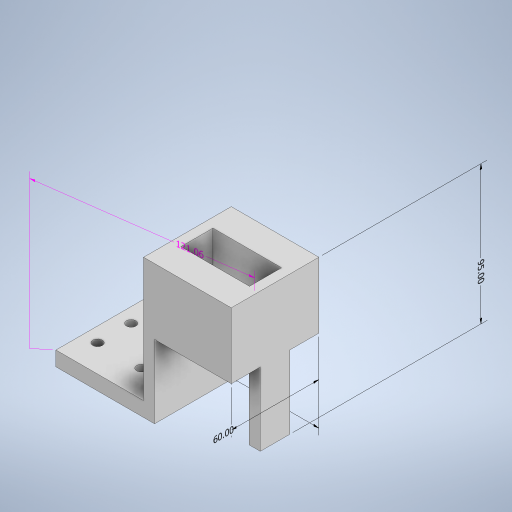
# Autodesk Inventor part: depth_camera_support_v2
Saved by Autodesk Inventor 2023 (Build 270158000, 158)
## iProperties
Created: 2023-05-27
Part Number: depth_camera_support_v2
Material: Genérico
Document SubType Name: Modeling
Designer: inigo
Density: 1 g/cm^3
Appearance: Valor por defecto
Author: inigo
Autodesk Inventor part; units mm, degrees
ref_plane "YZ Plane" through (0, 0, 0) normal (1, 0, 0) x (0, 1, 0)
ref_plane "XZ Plane" through (0, 0, 0) normal (0, 1, 0) x (-1, 0, 0)
ref_plane "XY Plane" through (0, 0, 0) normal (0, 0, 1) x (1, 0, 0)
sketch "Boceto2" plane through (0, 0, 0) normal (0, 1, 0) x (-1, 0, 0)
  line L0 (-30, 30) -> (30, 30)
  line L1 (30, 30) -> (30, -30)
  line L2 (30, -30) -> (-30, -30)
  line L3 (-30, -30) -> (-30, 30)
  line L4 (-30, 30) -> (30, -30) construction
  line L5 (30, 30) -> (-30, -30) construction
  point P0 (0, 0)
  dimension "d0" = 60
  dimension "d1" = 60
  constraints: 12 end point, 2 midpoint, 2 parallel, 1 horizontal, 1 perpendicular
  measures "d0" distance of L1.end L2.end
  measures "d1" distance of L0.end L1.end
extrude "Extrusión1" add sketch "Boceto2" along normal blind 55
sketch "Boceto3" plane through (30, 0, -30) normal (0, 0, -1) x (-1, 0, 0)
  line L0 (7.5, 50) -> (52.5, 50)
  line L1 (52.5, 50) -> (52.5, 0)
  line L2 (52.5, 0) -> (7.5, 0)
  line L3 (7.5, 0) -> (7.5, 50)
  line L4 (0, 0) -> (60, 0) projected
  point P0 (30, 0)
  dimension "d4" = 45
  dimension "d5" = 50
  dimension "d6" = 0
  constraints: 8 end point, 2 parallel, 1 horizontal, 1 perpendicular
  measures "d4" distance of L1.end L2.end
  measures "d5" distance of L0.end L1.end
  measures "d6" distance between parallel lines of L4 L2
extrude "Extrusión2" cut sketch "Boceto3" against normal blind 190
sketch "Boceto5" plane through (0, 0, 0) normal (0, 1, 0) x (-1, 0, 0)
  line L0 (30, -30) -> (30, 30) projected
  line L1 (30, 0) -> (60, 0)
  line L2 (90, 30) -> (30, 30)
  line L3 (30, 30) -> (30, -30)
  line L4 (30, -30) -> (90, -30)
  line L5 (90, -30) -> (90, 30)
  line L6 (90, 30) -> (30, -30) construction
  line L7 (30, 30) -> (90, -30) construction
  circle A0 centre (50, 11.5) radius 3.25
  circle A1 centre (50, -11.5) radius 3.25
  circle A2 centre (80, 11.5) radius 3.25
  circle A3 centre (80, -11.5) radius 3.25
  point P0 (0, 0)
  dimension "d16" = 30
  dimension "d17" = 60
  dimension "d18" = 60
  dimension "d19" = 6.5
  dimension "d20" = 20
  dimension "d21" = 18.5
  dimension "d22" = 23
  dimension "d23" = 6.5
  dimension "d24" = 30
  dimension "d25" = 18.5
  constraints: 14 end point, 4 centre point, 3 midpoint, 2 horizontal, 2 parallel, 2 symmetric about line, 1 perpendicular, 2 other
  measures "d16" distance of L1.start L1.end
  measures "d17" distance of L4.end L3.end
  measures "d18" distance of L3.end L2.end
  measures "d19" diameter of A0
  measures "d20" distance from line of L0 A0.centre
  measures "d21" distance from line of L2 A0.centre
  measures "d22" distance of A1.centre A0.centre
  measures "d23" diameter of A2
  measures "d24" distance of A0.centre A2.centre
  measures "d25" distance from line of L2 A2.centre
extrude "Extrusión4" add sketch "Boceto5" along normal blind 10
sketch "Boceto6" plane through (0, 55, 0) normal (0, 1, 0) x (1, 0, 0)
  line L0 (-30, 30) -> (-30, -30) projected
  line L1 (30, -30) -> (-30, -30)
  line L2 (-30, -30) -> (-30, 30)
  line L3 (-30, 30) -> (30, 30)
  line L4 (30, 30) -> (30, -30)
  line L5 (30, -30) -> (-30, 30) construction
  line L6 (-30, -30) -> (30, 30) construction
  point P0 (0, 0)
  dimension "d28" = 60
  constraints: 12 end point, 2 midpoint, 2 parallel, 1 horizontal, 1 perpendicular, 1 point on line
  measures "d28" distance of L1.end L2.end
extrude "Extrusión5" add sketch "Boceto6" along normal blind 40
sketch "Boceto7" plane through (0, 95, 0) normal (0, 1, 0) x (1, 0, 0)
  line L0 (-23.5, 11) -> (23.5, 11)
  line L1 (23.5, 11) -> (23.5, -11)
  line L2 (23.5, -11) -> (-23.5, -11)
  line L3 (-23.5, -11) -> (-23.5, 11)
  line L4 (-23.5, 11) -> (23.5, -11) construction
  line L5 (23.5, 11) -> (-23.5, -11) construction
  point P0 (0, 0)
  dimension "d31" = 47
  dimension "d32" = 22
  constraints: 12 end point, 2 midpoint, 2 parallel, 1 horizontal, 1 perpendicular
  measures "d31" distance of L1.end L2.end
  measures "d32" distance of L0.end L1.end
extrude "Extrusión6" cut sketch "Boceto7" against normal blind 43
sketch "Boceto8" plane through (-30, 0, 30) normal (-1, 0, 0) x (0, 0, 1)
  line L0 (-60, 55) -> (-44, 55) projected
  line L1 (0, 55) -> (-16, 55) projected
  line L2 (-44, 55) -> (-16, 55)
  line L3 (-41, 65) -> (-19, 65)
  line L4 (-19, 65) -> (-19, 55)
  line L5 (-19, 55) -> (-41, 55)
  line L6 (-41, 55) -> (-41, 65)
  line L7 (-41, 65) -> (-19, 55) construction
  line L8 (-19, 65) -> (-41, 55) construction
  line L9 (-16, 55) -> (-16, 95) projected
  line L10 (-44, 55) -> (-44, 95) projected
  point P0 (-30, 0)
  point P1 (-30, 60)
  point P2 (-41, 55)
  point P3 (-19, 55)
  point P4 (0, 95)
  point P5 (-60, 95)
  point P6 (-41, 60)
  dimension "d35" = 22
  dimension "d36" = 10
  dimension "d37" = 0
  dimension "d53" = 3
  dimension "d54" = 3
  constraints: 14 end point, 3 midpoint, 2 parallel, 1 collinear, 1 horizontal, 1 perpendicular
  measures "d35" distance of L4.end L5.end
  measures "d36" distance of L3.end L4.end
  measures "d37" distance between parallel lines of L5 L2
  measures "d53" distance between parallel lines of L9 L4
  measures "d54" distance from line of L10 point (-41, 60)
extrude "Extrusión7" cut sketch "Boceto8" against normal blind 10
ref_plane "Plano de trabajo1" through (30, 55, 0) normal (0, 0, -1) x (-1, 0, 0)
sketch "Boceto10" plane through (30, 55, 0) normal (0, 0, -1) x (-1, 0, 0)
  line L0 (60.12, -45) -> (60.12, 17.4198)
  line L1 (60.12, -45) -> (60.12, 13.5667)
  line L2 (60.12, -45) -> (137.1989, -45)
  line L3 (60.12, -19.9519) -> (80.5233, -61.6073)
  line L4 (120, -45) -> (60, -45) projected
  point P0 (30, -55)
  point P1 (72.3889, -45)
  dimension "d41" = 0
  constraints: 8 end point, 2 point on line
  measures "d41" distance between parallel lines of L4 L2
extrude "Extrusión8" add sketch "Boceto10" along normal mid plane 15
sketch "Boceto11" plane through (30, 0, 30) normal (1, 0, 0) x (0, 0, -1)
  line L0 (30, 0) -> (30, 50)
  line L1 (60, 50) -> (0, 50) projected
  line L2 (0, 0) -> (60, 0) projected
  line L3 (20, 50) -> (40, 50)
  line L4 (40, 50) -> (40, 0)
  line L5 (40, 0) -> (20, 0)
  line L6 (20, 0) -> (20, 50)
  line L7 (20, 50) -> (40, 0) construction
  line L8 (40, 50) -> (20, 0) construction
  line L9 (60, 0) -> (60, 95) projected
  line L10 (40, 50) -> (60, 50)
  line L11 (60, 50) -> (60, 0)
  line L12 (60, 0) -> (40, 0)
  line L13 (40, 0) -> (40, 50)
  line L14 (0, 0) -> (0, 95) projected
  line L15 (19.8706, 50) -> (0, 50)
  line L16 (0, 50) -> (0, 0)
  line L17 (0, 0) -> (19.8706, 0)
  line L18 (19.8706, 0) -> (19.8706, 50)
  point P0 (30, 25)
  dimension "d55" = 20
  constraints: 30 end point, 6 parallel, 4 midpoint, 3 horizontal, 3 perpendicular, 2 point on line
  measures "d55" distance of L4.end L5.end
extrude "Extrusión9" cut sketch "Boceto11" against normal blind 10 contours L4 L1 L9 L2 | L2 L14 L1 L18
